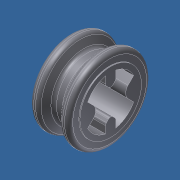
# Autodesk Inventor part: 4265C
Saved by Autodesk Inventor 2011 SP2 (Build 150553200, 553)
## iProperties
Company: Allseas Engineering BV
Created: 2011-12-01
Part Number: 4265C
Cost Center: 0 kg
Material: Steel
Document SubType Name: Modeling
Designer: PMe
Authority: 0 mm^3
Stock Number: =<Filenr>_<Document number>
Mass: 0.793025 g
Surface Area: 2.55466 cm^2
Volume: 0.101022 cm^3
Density: 7.85 g/cm^3
Act. Code: DW000
SaveDate: 2011-07-28
SaveTime: 18:32
FileName: Standard
TotalMass: 0 kg
TotalVolume: 0 mm^3
Subject: =<Title><TITLE 1_2> <TITLE 2_2>
Author: PMe
Autodesk Inventor part; units mm, degrees
ref_plane "YZ Plane" through (0, 0, 0) normal (1, 0, 0) x (0, 1, 0)
ref_plane "XZ Plane" through (0, 0, 0) normal (0, 1, 0) x (-1, 0, 0)
ref_plane "XY Plane" through (0, 0, 0) normal (0, 0, 1) x (1, 0, 0)
sketch "Sketch1" plane through (0, 0, 0) normal (0, 0, 1) x (1, 0, 0)
  line L0 (-2, 0) -> (2, 0)
  line L1 (-2, 0) -> (-2, 3)
  line L2 (-2, 3) -> (-1.9, 3)
  line L3 (0, 0) -> (0, 3) construction
  line L4 (-1.9, 3) -> (-1.9, 3.6)
  line L5 (-1.5, 4) -> (-1.3196, 4)
  line L6 (-0.9732, 3.8) -> (-0.6268, 3.2)
  line L7 (-0.2804, 3) -> (0, 3)
  arc A0 (-0.9732, 3.8) -> (-1.3196, 4) centre (-1.3196, 3.6) ccw
  arc A1 (-0.6268, 3.2) -> (-0.2804, 3) centre (-0.2804, 3.4) ccw
  arc A2 (-1.5, 4) -> (-1.9, 3.6) centre (-1.5, 3.6) ccw
  line L8 (2, 0) -> (2, 3)
  line L9 (2, 3) -> (1.9, 3)
  line L10 (1.9, 3) -> (1.9, 3.6)
  line L11 (1.5, 4) -> (1.3196, 4)
  line L12 (0.9732, 3.8) -> (0.6268, 3.2)
  line L13 (0.2804, 3) -> (0, 3)
  arc A3 (1.3196, 4) -> (0.9732, 3.8) centre (1.3196, 3.6) ccw
  arc A4 (0.2804, 3) -> (0.6268, 3.2) centre (0.2804, 3.4) ccw
  arc A5 (1.9, 3.6) -> (1.5, 4) centre (1.5, 3.6) ccw
  line L14 (-0.8, 3.5) -> (0.8, 3.5) construction
  dimension "d0" = 0.4
  dimension "d1" = 8
  dimension "d2" = 6
  dimension "d3" = 6
  dimension "d4" = 4
  dimension "d5" = 3.8
  dimension "d8" = 1.6
  dimension "d9" = 120
  constraints: 30 end point, 12 point on circle, 11 symmetric about line, 6 centre point, 6 tangent, 4 perpendicular, 3 midpoint, 2 equal radius, 2 horizontal, 1 coincident, 1 parallel, 3 other
  measures "d0" radius of A0
  measures "d1" diameter of L5 L0
  measures "d2" diameter of L7 L0
  measures "d3" diameter of L2 L0
  measures "d4" distance of L0.start L0.end
  measures "d5" distance between parallel lines of L10 L4
  measures "d8" distance of L14.start L14.end
  measures "d9" angle of L7 L6
revolve "Revolution1" add sketch "Sketch1" angle 360 about axis through (-2, 0, 0) along (1, 0, 0)
sketch "Sketch2" plane through (2, 0, 0) normal (1, 0, 0) x (0, 0, -1)
  circle A0 centre (0, 0) radius 2.5
  line L0 (2.2405, -1.1091) -> (1.6314, -0.5) construction
  line L1 (1.1314, 0) -> (1.6314, 0.5)
  line L2 (-2.2405, 1.1091) -> (-1.6314, 0.5) construction
  line L3 (-1.1314, 0) -> (-1.6314, -0.5)
  line L4 (-1.1091, -2.2405) -> (0, -1.1314)
  line L5 (0, -1.1314) -> (1.1091, -2.2405)
  line L6 (1.1091, 2.2405) -> (0, 1.1314)
  line L7 (0, 1.1314) -> (-1.1091, 2.2405)
  line L8 (-1.6314, -0.5) -> (-2.4495, -0.5)
  line L9 (-1.6314, 0.5) -> (-2.4495, 0.5)
  line L10 (1.6314, -0.5) -> (2.4495, -0.5)
  line L11 (1.6314, 0.5) -> (2.4495, 0.5)
  line L12 (-1.6314, -0.5) -> (-2.2405, -1.1091) construction
  line L13 (1.6314, -0.5) -> (1.1314, 0)
  line L14 (1.6314, 0.5) -> (2.2405, 1.1091) construction
  line L15 (-1.6314, 0.5) -> (-1.1314, 0)
  point P0 (0, 0)
  dimension "d11" = 5
  dimension "d12" = 1.6
  dimension "d13" = 1
  dimension "d14" = 1
  dimension "d15" = 1.5685
  dimension "d16" = 1.5685
  dimension "d17" = 1.6
  dimension "d18" = 1.6
  dimension "d19" = 1.6
  constraints: 32 end point, 11 perpendicular, 5 equal length, 5 parallel, 2 collinear, 1 coincident, 1 horizontal, 1 vertical alignment, 14 other
  measures "d12" distance between parallel lines of L2 L7
  measures "d13" distance between parallel lines of L9 L8
  measures "d14" distance between parallel lines of L11 L10
  measures "d15" distance of L4.start L4.end
  measures "d16" distance of L12.end L3.start
  measures "d17" distance between parallel lines of L6 L14
  measures "d18" distance between parallel lines of L5 L0
  measures "d19" distance between parallel lines of L12 L4
extrude "Extrusion1" cut sketch "Sketch2" against normal through all contours L11 L1 L13 L10 A0 L5 L4 L8 L3 L15 L9 L7 L6
fillet "Fillet1" radius 0.3 6 edges at (0, 0, 1.1314) (0, 0.5, 1.6314) (0, -0.5, 1.6314) (0, 0.5, -1.6314) (0, 0, -1.1314) (0, -0.5, -1.6314)
fillet "Fillet2" radius 0.8 2 edges at (0, -1.1314, 0) (0, 1.1314, 0)
equation "\"d3\" = d2"
equation "\"d14\" = d13"
equation "\"d16\" = d15"
equation "\"d17\" = d12"
equation "\"d18\" = d17"
equation "\"d19\" = d12"
body "Solid1"
